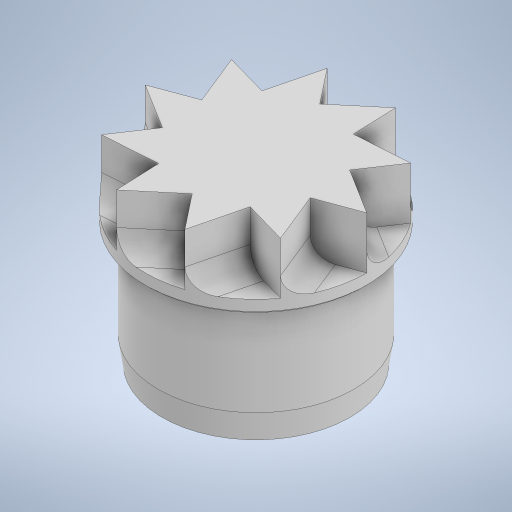
# Autodesk Inventor part: 7mm_uncorrected_thin
Saved by Autodesk Inventor 2023.1 (Build 271208000, 208)
## iProperties
Created: 2022-06-24
Part Number: 7mm_uncorrected_thin
Material: Générique
Document SubType Name: Modeling
Designer: Cyriaque
Density: 1 g/cm^3
Appearance: Par défaut
Author: Cyriaque
Autodesk Inventor part; units mm, degrees
ref_plane "YZ Plane" through (0, 0, 0) normal (1, 0, 0) x (0, 1, 0)
ref_plane "XZ Plane" through (0, 0, 0) normal (0, 1, 0) x (-1, 0, 0)
ref_plane "XY Plane" through (0, 0, 0) normal (0, 0, 1) x (1, 0, 0)
sketch "Esquisse1" plane through (0, 0, 0) normal (0, 1, 0) x (-1, 0, 0)
  circle A0 centre (0, 0) radius 3.4
  line L0 (2.7507, 1.9985) -> (2.0014, 0.8755)
  line L1 (2.0014, 0.8755) -> (3.4, 0)
  line L2 (0, 0) -> (3.747, 0)
  line L3 (1.1046, 1.8847) -> (2.7507, 1.9985)
  line L4 (1.0507, 3.2336) -> (1.1046, 1.8847)
  line L5 (-0.2142, 2.174) -> (1.0507, 3.2336)
  line L6 (-1.0507, 3.2336) -> (-0.2142, 2.174)
  line L7 (-1.4511, 1.6329) -> (-1.0507, 3.2336)
  line L8 (-2.7507, 1.9985) -> (-1.4511, 1.6329)
  line L9 (-2.1338, 0.4681) -> (-2.7507, 1.9985)
  line L10 (-3.4, 0) -> (-2.1338, 0.4681)
  line L11 (-2.0014, -0.8755) -> (-3.4, 0)
  line L12 (-2.7507, -1.9985) -> (-2.0014, -0.8755)
  line L13 (-1.1046, -1.8847) -> (-2.7507, -1.9985)
  line L14 (-1.0507, -3.2336) -> (-1.1046, -1.8847)
  line L15 (0.2142, -2.174) -> (-1.0507, -3.2336)
  line L16 (1.0507, -3.2336) -> (0.2142, -2.174)
  line L17 (1.4511, -1.6329) -> (1.0507, -3.2336)
  line L18 (2.7507, -1.9985) -> (1.4511, -1.6329)
  line L19 (2.1338, -0.4681) -> (2.7507, -1.9985)
  line L20 (3.4, 0) -> (2.1338, -0.4681)
  point P0 (-3.4, 0)
  dimension "d0" = 6.8
  dimension "d3" = 360
  dimension "d5" = 1.35
  dimension "d6" = 1.65
  constraints: 42 end point, 2 coincident, 2 point on circle, 1 centre point, 1 horizontal, 1 point on line, 51 other
  measures "d0" diameter of A0
  measures "d5" distance of L0.start L0.end
  measures "d6" distance of L0.end L1.end
extrude "Extrusion1" add sketch "Esquisse1" along normal blind 1.6 contours L20 L19 L18 L17 L16 L15 L14 L13 L12 L11 L10 L9 L8 L7 L6 L5 L4 L3 L0 L1
extrude "Extrusion2" add sketch "Esquisse1" against normal blind 0.4
sketch "Esquisse2" plane through (0, -0.4, 0) normal (0, -1, 0) x (1, 0, 0)
  circle A0 centre (0, 0) radius 3
  circle A1 centre (0, 0) radius 2.2
  dimension "d11" = 6
  dimension "d12" = 4.4
  constraints: 2 centre point, 2 coincident
  measures "d11" diameter of A0
  measures "d12" diameter of A1
extrude "Extrusion3" add sketch "Esquisse2" along normal blind 3.7
fillet "Congé1" radius 0.6 10 edges at (-2.4422, 0, -1.2333) (-1.2509, 0, -2.4333) (0.4183, 0, -2.7038) (1.9276, 0, -1.9416) (2.7007, 0, -0.4377) (2.4422, 0, 1.2333) (1.2509, 0, 2.4333) (-0.4183, 0, 2.7038) (-1.9276, 0, 1.9416) (-2.7007, 0, 0.4377)
chamfer "Chanfrein1" distance 0.8 angle 8 1 edges at (-3, -4.1, 0) measured on face at (2.9903, -2.8667, -0.2414)
chamfer "Chanfrein2" distance 0.075 angle 45 1 edges at (3.4, -0.4, 0)
